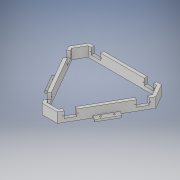
# Autodesk Inventor part: Stewart_Base
Saved by Autodesk Inventor 2018.1 (Build 221171000, 171)
## iProperties
Created: 2017-11-09
Part Number: Stewart_Base
Material: Generic
Document SubType Name: Modeling
Designer: sodie
Density: 1 g/cm^3
Appearance: Default
Author: sodie
Autodesk Inventor part; units mm, degrees
ref_plane "YZ Plane" through (0, 0, 0) normal (1, 0, 0) x (0, 1, 0)
ref_plane "XZ Plane" through (0, 0, 0) normal (0, 1, 0) x (-1, 0, 0)
ref_plane "XY Plane" through (0, 0, 0) normal (0, 0, 1) x (1, 0, 0)
sketch "Sketch1" plane through (0, 0, 0) normal (0, 0, 1) x (1, 0, 0)
  circle A0 centre (0, 0) radius 80
  line L0 (-61.2836, 51.423) -> (61.2836, 51.423)
  line L1 (75.1754, 27.3616) -> (13.8919, -78.7846)
  line L2 (-101.1421, 41.2372) -> (-14.8585, -108.2103)
  line L3 (101.142, 41.237) -> (14.8585, -108.2103)
  line L4 (-75.1754, 27.3616) -> (-13.8919, -78.7846)
  line L5 (-86.2836, 66.973) -> (-101.1421, 41.2372)
  line L6 (101.142, 41.237) -> (86.2836, 66.973)
  line L7 (-86.2836, 66.973) -> (86.2836, 66.973)
  line L8 (14.8585, -108.2103) -> (-14.8585, -108.2103)
  line L9 (90.6137, 74.473) -> (109.8022, 41.237)
  line L10 (109.8022, 41.237) -> (19.1887, -115.7103)
  line L11 (19.1887, -115.7103) -> (-19.1887, -115.7103)
  line L12 (-19.1887, -115.7103) -> (-109.8024, 41.2372)
  line L13 (-109.8024, 41.2372) -> (-90.6137, 74.473)
  line L14 (-90.6137, 74.473) -> (90.6137, 74.473)
  line L15 (-77.0024, -15.574) -> (-87.8277, -21.824)
  line L16 (-87.8277, -21.824) -> (-62.814, -65.149)
  line L17 (-62.814, -65.149) -> (-51.9887, -58.899)
  line L18 (-25.0137, 74.473) -> (-25.0137, 86.973)
  line L19 (-25.0137, 86.973) -> (25.0137, 86.973)
  line L20 (25.0137, 86.973) -> (25.0137, 74.473)
  line L21 (77.0022, -15.5743) -> (87.8275, -21.8243)
  line L22 (87.8275, -21.8243) -> (62.814, -65.149)
  line L23 (62.814, -65.149) -> (51.9887, -58.899)
  point P0 (-61.2836, 51.423)
  dimension "d0" = 160
  dimension "d9" = 61.2836
  dimension "d10" = 27.3616
  dimension "d11" = 51.423
  dimension "d12" = 75.1754
  dimension "d15" = 78.7846
  dimension "d16" = 13.8918
  dimension "d17" = 13.8918
  dimension "d18" = 78.7846
  dimension "d19" = 27.3616
  dimension "d20" = 75.1754
  dimension "d21" = 61.2836
  dimension "d22" = 51.423
  dimension "d73" = 15.55
  dimension "d74" = 15.55
  dimension "d81" = 25
  dimension "d82" = 120
  dimension "d83" = 29.7171
  dimension "d86" = 29.7171
  dimension "d87" = 25
  dimension "d88" = 25.736
  dimension "d89" = 7.5
  dimension "d93" = 29.3301
  dimension "d294" = 12.5
  dimension "d295" = 65.6
  dimension "d296" = 65.6
  dimension "d297" = 50.0274
  dimension "d298" = 65.6
  dimension "d299" = 65.6
  dimension "d300" = 12.5
  dimension "d301" = 65.6
  dimension "d302" = 65.6
  dimension "d303" = 12.5
  constraints: 48 end point, 7 perpendicular, 6 point on line, 2 coincident, 2 horizontal, 2 parallel, 1 centre point, 1 vertical, 5 other
  measures "d0" diameter of A0
  measures "d9" horizontal distance of point (0, 0) point (-61.284, 51.423)
  measures "d10" vertical distance of point (0, 0) L4.start
  measures "d11" vertical distance of point (0, 0) point (-61.284, 51.423)
  measures "d12" horizontal distance of point (0, 0) L4.start
  measures "d15" vertical distance of point (0, 0) L4.end
  measures "d16" horizontal distance of point (0, 0) L4.end
  measures "d17" horizontal distance of point (0, 0) L1.end
  measures "d18" vertical distance of point (0, 0) L1.end
  measures "d19" vertical distance of point (0, 0) L1.start
  measures "d20" horizontal distance of point (0, 0) L1.start
  measures "d21" horizontal distance of point (0, 0) point (61.284, 51.423)
  measures "d22" vertical distance of point (0, 0) point (61.284, 51.423)
  measures "d73" distance between parallel lines of L1 L3
  measures "d74" distance between parallel lines of L2 L4
  measures "d81" horizontal distance of L5.start point (-61.284, 51.423)
  measures "d82" angle of L2 L5
  measures "d83" distance of L5.start L2.start
  measures "d86" distance of L3.end L2.end
  measures "d87" horizontal distance of L6.end point (61.284, 51.423)
  measures "d88" vertical distance of L3.start L6.end
  measures "d89" distance between parallel lines of L7 L14
  measures "d93" horizontal distance of point (-61.284, 51.423) L13.end
  measures "d294" distance between parallel lines of L12 L16
  measures "d295" distance from line of L12.end L15
  measures "d296" distance from line of L11.end L17
  measures "d297" distance of L15.end L16.end
  measures "d298" distance from line of L13.end L18
  measures "d299" distance from line of L9.start L20
  measures "d300" distance between parallel lines of L14 L19
  measures "d301" distance from line of L10.end L23
  measures "d302" distance from line of L9.end L21
  measures "d303" distance between parallel lines of L10 L22
extrude "Extrusion12" add sketch "Sketch1" along normal blind 25 contours L3 L6 L7 A0 L14 L9 L10 | A0 L10 L3 | L7 A0 L14 | A0 L10 L11 L12 L2 L8 L3 | L7 L5 L2 A0 L12 L13 L14 | A0 L12 L2
sketch "Sketch11" plane through (109.8022, 41.237, 25) normal (0.8660254, -0.5, 0) x (0, 0, -1)
  line L0 (25, 0) -> (25, -181.2271) projected
  line L1 (25, -90.6134) -> (-4.9231, -90.6134)
  line L2 (-1, -168.7974) -> (16.3, -168.7974)
  line L3 (16.3, -168.7974) -> (16.3, -145.4974)
  line L4 (16.3, -145.4974) -> (-1, -145.4974)
  line L5 (-1, -145.4974) -> (-1, -168.7974)
  line L6 (0, -181.2271) -> (0, 0) projected
  line L7 (-1, -35.7294) -> (16.3, -35.7294)
  line L8 (16.3, -35.7294) -> (16.3, -12.4294)
  line L9 (16.3, -12.4294) -> (-1, -12.4294)
  line L10 (-1, -12.4294) -> (-1, -35.7294)
  point P0 (10, -37.9294)
  point P1 (10, -29.3294)
  point P2 (10, -10.2294)
  point P3 (10, -143.2974)
  point P4 (10, -151.8974)
  point P5 (10, -170.9974)
  dimension "d223" = 8.6
  dimension "d224" = 19.1
  dimension "d226" = 61.284
  dimension "d228" = 61.284
  dimension "d229" = 8.6
  dimension "d230" = 19.1
  dimension "d271" = 1
  dimension "d272" = 2.2
  dimension "d273" = 2.2
  dimension "d274" = 6.3
  dimension "d275" = 1
  dimension "d276" = 6.3
  dimension "d277" = 2.2
  dimension "d278" = 2.2
  dimension "d293" = 10
  constraints: 18 end point, 4 parallel, 3 horizontal, 3 symmetric about line, 2 perpendicular, 2 vertical alignment
  measures "d223" distance of point (10, -29.329) point (10, -37.929)
  measures "d224" distance of point (10, -10.229) point (10, -29.329)
  measures "d226" vertical distance of L1.start point (10, -29.329)
  measures "d228" distance from line of L1 point (10, -151.897)
  measures "d229" distance of point (10, -151.897) point (10, -143.297)
  measures "d230" distance of point (10, -151.897) point (10, -170.997)
  measures "d271" distance between parallel lines of L6 L5
  measures "d272" distance from line of point (10, -170.997) L2
  measures "d273" distance from line of point (10, -143.297) L4
  measures "d274" distance from line of point (10, -143.297) L3
  measures "d275" distance between parallel lines of L6 L10
  measures "d276" distance from line of point (10, -37.929) L8
  measures "d277" distance from line of L7 point (10, -37.929)
  measures "d278" distance from line of point (10, -10.229) L9
  measures "d293" distance from line of L6 point (10, -10.229)
sketch "Sketch12" plane through (-90.6137, 74.473, 0) normal (0, 1, 0) x (1, 0, 0)
  line L0 (0, 0) -> (181.2274, 0) projected
  line L1 (90.6137, 0) -> (90.6137, -25.6857)
  line L2 (176.8972, 0) -> (4.3301, 0) projected
  line L3 (145.4977, -26) -> (168.7977, -26)
  line L4 (168.7977, -26) -> (168.7977, -8.7)
  line L5 (168.7977, -8.7) -> (145.4977, -8.7)
  line L6 (145.4977, -8.7) -> (145.4977, -26)
  line L7 (181.2274, -25) -> (0, -25) projected
  line L8 (35.7297, -26) -> (12.4297, -26)
  line L9 (12.4297, -26) -> (12.4297, -8.7)
  line L10 (12.4297, -8.7) -> (35.7297, -8.7)
  line L11 (35.7297, -8.7) -> (35.7297, -26)
  point P0 (170.9977, -15)
  point P1 (151.8977, -15)
  point P2 (143.2977, -15)
  point P3 (10.2297, -15)
  point P4 (29.3297, -15)
  point P5 (37.9297, -15)
  point P6 (157.1477, -26)
  dimension "d212" = 8.6
  dimension "d213" = 19.1
  dimension "d214" = 61.284
  dimension "d238" = 8.6
  dimension "d239" = 19.1
  dimension "d240" = 61.284
  dimension "d257" = 2.2
  dimension "d258" = 2.2
  dimension "d260" = 6.3
  dimension "d264" = 1
  dimension "d265" = 10
  dimension "d266" = 10
  dimension "d267" = 2.2
  dimension "d268" = 2.2
  dimension "d269" = 6.3
  dimension "d270" = 1
  constraints: 18 end point, 4 parallel, 3 perpendicular, 3 symmetric about line, 2 horizontal, 2 horizontal alignment, 1 midpoint
  measures "d212" distance of point (143.298, -15) point (151.898, -15)
  measures "d213" distance of point (151.898, -15) point (170.998, -15)
  measures "d214" horizontal distance of L1.start point (151.898, -15)
  measures "d238" distance of point (37.93, -15) point (29.33, -15)
  measures "d239" distance of point (29.33, -15) point (10.23, -15)
  measures "d240" horizontal distance of L1.start point (29.33, -15)
  measures "d257" distance from line of point (143.298, -15) L6
  measures "d258" distance from line of point (170.998, -15) L4
  measures "d260" distance from line of point (170.998, -15) L5
  measures "d264" distance between parallel lines of L7 L3
  measures "d265" distance from line of L7 point (143.298, -15)
  measures "d266" distance from line of L7 point (37.93, -15)
  measures "d267" distance from line of point (37.93, -15) L11
  measures "d268" distance from line of L9 point (10.23, -15)
  measures "d269" distance from line of point (37.93, -15) L10
  measures "d270" distance between parallel lines of L7 L8
hole "Hole8" at (52.684, 74.473, 15) at (80.384, 74.473, 15) at (-52.684, 74.473, 15) at (-80.384, 74.473, 15) direction (0, -1, 0) diameter 2 depth 10 tip angle 118
hole "Hole9" at (24.3035, -106.8511, 15) at (38.1535, -82.8622, 15) at (90.8375, 8.3892, 15) at (104.6875, 32.3781, 15) direction (-0.8660254, 0.5, 0) diameter 2 depth 10 tip angle 118
sketch "Sketch13" plane through (-19.1887, -115.7103, 0) normal (-0.8660254, -0.5, 0) x (0, 0, 1)
  line L0 (0, 90.6137) -> (30.0309, 90.6137)
  line L1 (0, 0) -> (0, 181.2274) projected
  line L2 (26, 168.7977) -> (8.7, 168.7977)
  line L3 (8.7, 168.7977) -> (8.7, 145.4977)
  line L4 (8.7, 145.4977) -> (26, 145.4977)
  line L5 (26, 145.4977) -> (26, 168.7977)
  line L6 (25, 181.2274) -> (25, 0) projected
  line L7 (26, 35.7297) -> (8.7, 35.7297)
  line L8 (8.7, 35.7297) -> (8.7, 12.4297)
  line L9 (8.7, 12.4297) -> (26, 12.4297)
  line L10 (26, 12.4297) -> (26, 35.7297)
  point P0 (15, 170.9977)
  point P1 (15, 151.8977)
  point P2 (15, 143.2977)
  point P3 (15, 10.2297)
  point P4 (15, 29.3297)
  point P5 (15, 37.9297)
  dimension "d242" = 19.1
  dimension "d243" = 8.6
  dimension "d244" = 61.284
  dimension "d246" = 8.6
  dimension "d247" = 19.1
  dimension "d248" = 61.284
  dimension "d281" = 2.2
  dimension "d282" = 2.2
  dimension "d283" = 1
  dimension "d284" = 6.3
  dimension "d285" = 10
  dimension "d286" = 10
  dimension "d287" = 1
  dimension "d288" = 2.2
  dimension "d289" = 2.2
  dimension "d290" = 6.3
  constraints: 18 end point, 4 parallel, 3 horizontal, 3 symmetric about line, 2 perpendicular, 2 vertical alignment
  measures "d242" distance of point (15, 151.898) point (15, 170.998)
  measures "d243" distance of point (15, 143.298) point (15, 151.898)
  measures "d244" distance from line of L0 point (15, 151.898)
  measures "d246" distance of point (15, 29.33) point (15, 37.93)
  measures "d247" distance of point (15, 29.33) point (15, 10.23)
  measures "d248" distance from line of L0 point (15, 29.33)
  measures "d281" distance from line of point (15, 170.998) L2
  measures "d282" distance from line of point (15, 143.298) L4
  measures "d283" distance between parallel lines of L6 L5
  measures "d284" distance from line of point (15, 143.298) L3
  measures "d285" distance from line of L6 point (15, 170.998)
  measures "d286" distance from line of L6 point (15, 37.93)
  measures "d287" distance between parallel lines of L6 L10
  measures "d288" distance from line of point (15, 37.93) L7
  measures "d289" distance from line of point (15, 10.23) L9
  measures "d290" distance from line of point (15, 37.93) L8
hole "Hole10" at (-104.6875, 32.3781, 15) at (-90.8375, 8.3892, 15) at (-38.1535, -82.8622, 15) at (-24.3035, -106.8511, 15) direction (0.8660254, 0.5, 0) diameter 2 depth 10 tip angle 118
extrude "Extrusion13" cut sketch "Sketch12" against normal blind 10
extrude "Extrusion14" cut sketch "Sketch11" against normal blind 10
extrude "Extrusion15" cut sketch "Sketch13" against normal blind 10
extrude "Extrusion16" add sketch "Sketch1" along normal blind 5 contours L20 L14 L18 A0 | A0 L18 L19 L20 | L21 L22 L23 A0 | A0 L23 L10 L21 | L17 L16 L15 A0 | A0 L15 L12 L17
sketch "Sketch14" plane through (0, 0, 5) normal (0, 0, 1) x (1, 0, 0)
  line L0 (62.814, -65.149) -> (87.8275, -21.8243) projected
  line L1 (51.9887, -58.899) -> (62.814, -65.149) projected
  line L2 (87.8275, -21.8243) -> (77.0022, -15.5743) projected
  point P0 (0, 0)
  point P1 (63.4348, -51.0737)
  point P2 (75.9484, -29.3996)
  dimension "d306" = 6.5
  dimension "d307" = 6.5
  dimension "d308" = 12.5
  dimension "d309" = 12.5
  measures "d306" distance from line of L0 point (63.435, -51.074)
  measures "d307" distance from line of L0 point (75.948, -29.4)
  measures "d308" distance from line of L1 point (63.435, -51.074)
  measures "d309" distance from line of L2 point (75.948, -29.4)
hole "Hole11" at (63.4348, -51.0737, 5) at (75.9484, -29.3996, 5) direction (0, 0, -1) diameter 4.5 depth 5
sketch "Sketch15" plane through (0, 0, 5) normal (0, 0, 1) x (1, 0, 0)
  line L0 (-87.8277, -21.824) -> (-62.814, -65.149) projected
  line L1 (-62.814, -65.149) -> (-51.9887, -58.899) projected
  line L2 (-77.0024, -15.574) -> (-87.8277, -21.824) projected
  point P0 (0, 0)
  point P1 (-75.9485, -29.3993)
  point P2 (-63.4348, -51.0737)
  dimension "d317" = 6.5
  dimension "d318" = 6.5
  dimension "d319" = 12.5
  dimension "d320" = 12.5
  measures "d317" distance from line of L0 point (-75.949, -29.399)
  measures "d318" distance from line of L0 point (-63.435, -51.074)
  measures "d319" distance from line of L1 point (-63.435, -51.074)
  measures "d320" distance from line of L2 point (-75.949, -29.399)
hole "Hole12" at (-75.9485, -29.3993, 5) at (-63.4348, -51.0737, 5) direction (0, 0, -1) diameter 4.5 depth 5
sketch "Sketch16" plane through (0, 0, 5) normal (0, 0, 1) x (1, 0, 0)
  line L0 (-25.0137, 86.973) -> (-25.0137, 74.473) projected
  line L1 (25.0137, 74.473) -> (25.0137, 86.973) projected
  line L2 (25.0137, 86.973) -> (-25.0137, 86.973) projected
  point P0 (0, 0)
  point P1 (-12.5137, 80.473)
  point P2 (12.5137, 80.473)
  dimension "d328" = 12.5
  dimension "d329" = 12.5
  dimension "d330" = 6.5
  dimension "d331" = 6.5
  measures "d328" distance from line of L0 point (-12.514, 80.473)
  measures "d329" distance from line of L1 point (12.514, 80.473)
  measures "d330" distance from line of L2 point (-12.514, 80.473)
  measures "d331" distance from line of L2 point (12.514, 80.473)
hole "Hole13" at (-12.5137, 80.473, 5) at (12.5137, 80.473, 5) direction (0, 0, -1) diameter 4.5 depth 5
body "Solid4"
